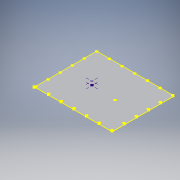
# Autodesk Inventor part: RFT 8x10 Cover-alt-base_092717
Saved by Autodesk Inventor 2017 (Build 210142000, 142)
## iProperties
Created: 2014-01-15
Part Number: RFT 8x10 Cover-alt-base_092717
Material: Aluminum 6061
Document SubType Name: Modeling
Designer: rtreacy
Density: 1 g/cm^3
Appearance: Aluminum - Flat
Author: rtreacy
Autodesk Inventor part; units mm, degrees
ref_plane "YZ Plane" through (0, 0, 0) normal (1, 0, 0) x (0, 1, 0)
ref_plane "XZ Plane" through (0, 0, 0) normal (0, 1, 0) x (-1, 0, 0)
ref_plane "XY Plane" through (0, 0, 0) normal (0, 0, 1) x (1, 0, 0)
sketch "Sketch1" plane through (0, 0, 0) normal (0, 1, 0) x (-1, 0, 0)
  line L0 (-82.5293, 92.3687) -> (171.4707, 92.3687)
  line L1 (171.4707, 92.3687) -> (171.4707, -110.8313)
  line L2 (171.4707, -110.8313) -> (-82.5293, -110.8313)
  line L3 (-82.5293, -110.8313) -> (-82.5293, 92.3687)
  point P0 (0, 0)
  dimension "d0" = 254
  dimension "d3" = 203.2
  constraints: 8 end point, 2 parallel, 1 horizontal, 1 perpendicular
  measures "d0" distance of L0.start L0.end
  measures "d3" distance of L0.end L1.end
extrude "Extrusion1" add sketch "Sketch1" along normal blind 1.524
sketch "Sketch2" plane through (0, 1.524, 0) normal (0, 1, 0) x (1, 0, 0)
  point P0 (0, 0)
  point P1 (-169.0958, 108.4564)
  point P2 (-171.4707, 110.8313)
  point P3 (82.5293, -92.3687)
  point P4 (80.1544, -89.9938)
  dimension "d13" = 2.3749
  dimension "d14" = 2.3749
  dimension "d21" = 2.3749
  dimension "d22" = 2.3749
  measures "d13" horizontal distance of point (-171.471, 110.831) point (-169.096, 108.456)
  measures "d14" horizontal distance of point (-171.471, 110.831) point (-169.096, 108.456)
  measures "d21" horizontal distance of point (82.529, -92.369) point (80.154, -89.994)
  measures "d22" horizontal distance of point (82.529, -92.369) point (80.154, -89.994)
hole "Hole1" at (-169.0958, 1.524, -108.4564) direction (0, -1, 0) diameter 2.4384 depth 25.4 tip angle 118 countersink diameter 4.064 countersink angle 82
pattern_linear "Rectangular Pattern1" count 7 spacing 41.529 along (1, 0, 0) of "Hole1"
pattern_linear "Rectangular Pattern2" count 5 spacing 39.6748 along (0, 0, 1) of "Hole1"
hole "Hole2" at (80.1544, 1.524, 89.9938) direction (0, -1, 0) diameter 2.4384 depth 25.4 tip angle 118 countersink diameter 4.064 countersink angle 82
pattern_linear "Rectangular Pattern3" count 5 spacing 39.6748 along (0, 0, -1) of "Hole2"
pattern_linear "Rectangular Pattern4" count 7 spacing 41.529 along (-1, 0, 0) of "Hole2"
sketch "Sketch3" plane through (0, 1.524, 0) normal (0, 1, 0) x (1, 0, 0)
  circle A0 centre (-169.0196, -89.9938) radius 2.032 projected
  circle A1 centre (-127.4906, -89.9938) radius 2.032 projected
  circle A2 centre (-85.9616, -89.9938) radius 2.032 projected
  circle A3 centre (-44.4326, -89.9938) radius 2.032 projected
  circle A4 centre (-2.9036, -89.9938) radius 2.032 projected
  circle A5 centre (38.6254, -89.9938) radius 2.032 projected
  circle A6 centre (80.1544, 68.7054) radius 2.032 projected
  circle A7 centre (80.1544, 29.0306) radius 2.032 projected
  circle A8 centre (80.1544, -10.6442) radius 2.032 projected
  circle A9 centre (80.1544, -50.319) radius 2.032 projected
  circle A10 centre (80.1544, -89.9938) radius 2.032 projected
  circle A11 centre (-169.0958, -50.2428) radius 2.032 projected
  circle A12 centre (-169.0958, -10.568) radius 2.032 projected
  circle A13 centre (-169.0958, 29.1068) radius 2.032 projected
  circle A14 centre (-169.0958, 68.7816) radius 2.032 projected
  circle A15 centre (80.0782, 108.4564) radius 2.032 projected
  circle A16 centre (38.5492, 108.4564) radius 2.032 projected
  circle A17 centre (-2.9798, 108.4564) radius 2.032 projected
  circle A18 centre (-44.5088, 108.4564) radius 2.032 projected
  circle A19 centre (-86.0378, 108.4564) radius 2.032 projected
  circle A20 centre (-127.5668, 108.4564) radius 2.032 projected
  circle A21 centre (-169.0958, 108.4564) radius 2.032 projected
  line L0 (-171.4707, -92.3687) -> (82.5293, -92.3687) projected
  line L1 (82.5293, -92.3687) -> (82.5293, 110.8313) projected
  line L2 (82.5293, 110.8313) -> (-171.4707, 110.8313) projected
  line L3 (-171.4707, 110.8313) -> (-171.4707, -92.3687) projected
  point P0 (0, 0)
sketch "Sketch6" plane through (0, 1.524, 0) normal (0, 1, 0) x (1, 0, 0)
  circle A0 centre (-169.0196, -89.9938) radius 2.032 projected
  circle A1 centre (-127.4906, -89.9938) radius 2.032 projected
  circle A2 centre (-85.9616, -89.9938) radius 2.032 projected
  circle A3 centre (-44.4326, -89.9938) radius 2.032 projected
  circle A4 centre (-2.9036, -89.9938) radius 2.032 projected
  circle A5 centre (38.6254, -89.9938) radius 2.032 projected
  circle A6 centre (80.1544, 68.7054) radius 2.032 projected
  circle A7 centre (80.1544, 29.0306) radius 2.032 projected
  circle A8 centre (80.1544, -10.6442) radius 2.032 projected
  circle A9 centre (80.1544, -50.319) radius 2.032 projected
  circle A10 centre (80.1544, -89.9938) radius 2.032 projected
  circle A11 centre (-169.0958, -50.2428) radius 2.032 projected
  circle A12 centre (-169.0958, -10.568) radius 2.032 projected
  circle A13 centre (-169.0958, 29.1068) radius 2.032 projected
  circle A14 centre (-169.0958, 68.7816) radius 2.032 projected
  circle A15 centre (80.0782, 108.4564) radius 2.032 projected
  circle A16 centre (38.5492, 108.4564) radius 2.032 projected
  circle A17 centre (-2.9798, 108.4564) radius 2.032 projected
  circle A18 centre (-44.5088, 108.4564) radius 2.032 projected
  circle A19 centre (-86.0378, 108.4564) radius 2.032 projected
  circle A20 centre (-127.5668, 108.4564) radius 2.032 projected
  circle A21 centre (-169.0958, 108.4564) radius 2.032 projected
  line L0 (-171.4707, -92.3687) -> (82.5293, -92.3687) projected
  line L1 (82.5293, -92.3687) -> (82.5293, 110.8313) projected
  line L2 (82.5293, 110.8313) -> (-171.4707, 110.8313) projected
  line L3 (-171.4707, 110.8313) -> (-171.4707, -92.3687) projected
  point P0 (0, 0)
sketch "Sketch7" plane through (0, 1.524, 0) normal (0, 1, 0) x (1, 0, 0)
  point P0 (0, 0)
  point P1 (-80.9959, 5.2689)
  point P2 (-93.6959, 17.9689)
  point P3 (-80.9959, 5.2689)
  point P4 (-171.4707, -92.3687)
  dimension "d50" = 110.3376
  dimension "d51" = 97.6376
  dimension "d52" = 77.7748
  dimension "d53" = 90.4748
  constraints: 1 coincident
  measures "d50" vertical distance of point (-171.471, -92.369) point (-93.696, 17.969)
  measures "d51" vertical distance of point (-171.471, -92.369) point (-80.996, 5.269)
  measures "d52" horizontal distance of point (-171.471, -92.369) point (-93.696, 17.969)
  measures "d53" horizontal distance of point (-171.471, -92.369) point (-80.996, 5.269)
hole "Hole3" at (-93.6959, 1.524, -17.9689) direction (0, -1, 0) diameter 3.2512 depth 1.524 tip angle 118 countersink diameter 5.8928 countersink angle 82
hole "Hole4" at (-80.9959, 1.524, -5.2689) direction (0, -1, 0) diameter 3.2512 depth 25.4 tip angle 118 countersink diameter 5.8928 countersink angle 82
body "Solid1"
